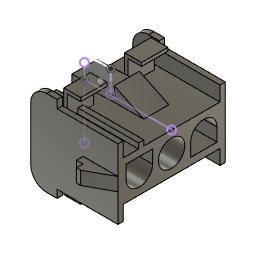
MLX_MF3_Connector_Mount (Autodesk Fusion 360 archive; units mm, degrees)
design "MLX Connector"
Autodesk Fusion 360 part; units mm, degrees
sketch "Sketch1" plane through (0, 0, 0) normal (1, 0, 0) x (0, 1, 0) in component "MLX Female Connector"
  line L0 (-10.15, 3.8) -> (-9.15, 3.8) construction
  line L1 (-9.15, -3.8) -> (-10.15, -3.8) construction
  line L2 (-10.15, -3.8) -> (-10.15, 3.8)
  line L3 (-10.15, 3.8) -> (-10.15, 6.6)
  line L4 (-10.15, 6.6) -> (-9.15, 6.6)
  line L5 (-9.15, 6.6) -> (-9.15, 3.8)
  line L6 (-10.15, -3.8) -> (-10.15, -6.6)
  line L7 (-10.15, -6.6) -> (-9.15, -6.6)
  line L8 (-9.15, -6.6) -> (-9.15, -3.8)
  line L9 (0, 3.8) -> (0, -3.8) construction
  line L10 (0, -3.8) -> (-9.15, -3.8)
  line L11 (-6.25, 3.8) -> (-5.25, 3.8)
  arc A0 (0, 2.5) -> (0, -2.5) centre (0, 0) ccw
  arc A1 (-8.6, 0) -> (-3.6, 0) centre (-6.1, 0) ccw
  line L12 (-3.6, 0) -> (-3.6, 2.5)
  line L13 (-3.6, 2.5) -> (-8.6, 2.5)
  line L14 (-8.6, 2.5) -> (-8.6, 0)
  line L15 (-6.25, 3.8) -> (-6.25, 4.8)
  line L16 (-6.25, 4.8) -> (-5.25, 4.8)
  line L17 (-5.25, 4.8) -> (-5.25, 3.8)
  line L18 (-5.25, 3.8) -> (0, 3.8)
  line L19 (-9.15, 3.8) -> (-6.25, 3.8)
  line L20 (5.25, 3.8) -> (0, 3.8)
  line L21 (6.25, 3.8) -> (5.25, 3.8)
  line L22 (0, -3.8) -> (9.15, -3.8)
  line L23 (9.15, -6.6) -> (9.15, -3.8)
  line L24 (10.15, -6.6) -> (9.15, -6.6)
  line L25 (10.15, -3.8) -> (10.15, -6.6)
  line L26 (10.15, -3.8) -> (10.15, 3.8)
  line L27 (10.15, 6.6) -> (9.15, 6.6)
  line L28 (9.15, 6.6) -> (9.15, 3.8)
  line L29 (10.15, 3.8) -> (10.15, 6.6)
  line L30 (9.15, 3.8) -> (6.25, 3.8)
  arc A2 (0, -2.5) -> (0, 2.5) centre (0, 0) ccw
  arc A3 (8.6, 0) -> (3.6, 0) centre (6.1, 0) ccw
  line L31 (3.6, 0) -> (3.6, -2.5)
  line L32 (3.6, -2.5) -> (8.6, -2.5)
  line L33 (8.6, -2.5) -> (8.6, 0)
  point P0 (10.15, 0)
  dimension "d4" = 7.6
  dimension "d5" = 1
  dimension "d6" = 2.8
  dimension "d7" = 10.15
  dimension "d8" = 2.5
  dimension "d9" = 2.5
  dimension "d10" = 6.1
  dimension "d11" = 1
  dimension "d12" = 1
  dimension "d13" = 4.9
  dimension "d15" = 6.1
  constraint horizontal L0
  constraint horizontal L1
  constraint vertical L2
  constraint vertical A0.centre L9.start
  constraint horizontal A0.centre P0
  constraint perpendicular L0 L3
  constraint perpendicular L3 L4
  constraint perpendicular L4 L5
  constraint perpendicular L1 L6
  constraint perpendicular L6 L7
  constraint perpendicular L1 L8
  constraint vertical L0.end L1.start
  constraint equal L3 L6
  constraint coincident L9.start L18.end
  constraint vertical L9
  constraint midpoint A0.centre L9
  constraint horizontal L10
  constraint horizontal L11
  constraint coincident L9 A0.end
  constraint coincident L9 A0.start
  constraint coincident A0.centre A2.centre
  constraint horizontal A1.start A1.end
  constraint horizontal A1.end A1.centre
  constraint horizontal A0.centre A1.centre
  constraint tangent A1 L12
  constraint perpendicular L12 L13
  constraint tangent A1 L14
  constraint tangent A0 L13
  constraint perpendicular L11 L15
  constraint perpendicular L15 L16
  constraint perpendicular L11 L17
  constraint horizontal L18
  constraint horizontal L19
  constraint symmetric L0.start L9 L26.end
  constraint symmetric L1.end L9 L25.start
  constraint symmetric L18.end L9 L20.end
  constraint symmetric L3.end L9 L27.start
  constraint symmetric L4.end L9 L27.end
  constraint symmetric L0.end L9 L28.end
  constraint symmetric L6.end L9 L24.start
  constraint symmetric L7.end L9 L23.start
  constraint symmetric L1.start L9 L22.end
  constraint symmetric L10.start L9 L22.start
  constraint symmetric L9 A0.start A2.end
  constraint symmetric L9 A0.end A2.start
  constraint symmetric L9 A0 A2
  constraint symmetric L9 L11.start L21.start
  constraint symmetric L9 L11.end L20.start
  constraint vertical L31
  constraint perpendicular L31 L32
  constraint perpendicular L32 L33
  constraint equal A1 A3
  constraint equal L12 L31
  constraint equal L31 L33
  constraint equal L13 L32
  constraint horizontal A1.centre A3.centre
  measures "d4" distance of L0.start L1.end
  measures "d5" distance of L3.end L4.end
  measures "d6" distance of L0.start L3.end
  measures "d7" distance of L2 L9
  measures "d8" radius of A0
  measures "d9" radius of A1
  measures "d10" horizontal distance of A0.centre A1.centre
  measures "d11" distance of L15.end L16.end
  measures "d12" distance of L11.start L15.end
  measures "d13" distance of L3 L17
  measures "d15" distance of A0.centre A3.centre
extrude "Extrude1" add sketch "Sketch1" along normal mid plane 16.5 in component "MLX Female Connector"
sketch "Sketch2" plane through (0, 0, 0) normal (0, 1, 0) x (1, 0, 0) in component "MLX Female Connector"
  line L0 (-8.25, -3.8) -> (8.25, -3.8)
  line L1 (8.25, -3.8) -> (-8.25, -3.8)
  line L2 (-8.25, -3.8) -> (-8.25, -5.9)
  line L3 (-8.25, -5.9) -> (0.001, -6.3012)
  line L4 (0.001, -6.3012) -> (-0.2312, -8)
  line L5 (-0.2312, -8) -> (5.35, -5.3)
  line L6 (5.35, -5.3) -> (0.001, -5.3)
  line L7 (0.001, -5.3) -> (-7.25, -4.9474)
  line L8 (-7.25, -4.9474) -> (-7.25, -3.8)
  line L9 (-8.25, 0) -> (8.25, 0) construction
  line L10 (-8.25, 3.8) -> (-8.25, 5.9)
  line L11 (-8.25, 5.9) -> (0.001, 6.3012)
  line L12 (0.001, 6.3012) -> (-0.2312, 8)
  line L13 (-0.2312, 8) -> (5.35, 5.3)
  line L14 (5.35, 5.3) -> (0.001, 5.3)
  line L15 (0.001, 5.3) -> (-7.25, 4.9474)
  line L16 (-7.25, 4.9474) -> (-7.25, 3.8)
  line L17 (8.25, 3.8) -> (-8.25, 3.8)
  dimension "d19" = 13.6
  dimension "d20" = 2.1
  dimension "d21" = 1
  dimension "d22" = 1
  dimension "d25" = 85
  dimension "d26" = 6.2
  dimension "d29" = 1.5
  dimension "d30" = 4.2
  constraint coincident L0.start L1.end
  constraint perpendicular L0 L2
  constraint parallel L3 L7
  constraint coincident L1 L8.end
  constraint perpendicular L1 L8
  constraint horizontal L6
  constraint vertical L3.end L6.end
  constraint parallel L0 L9
  constraint vertical L0.end L9.end
  constraint vertical L0.start L9.start
  constraint coincident origin L9
  constraint symmetric L0.start L9 L10.start
  constraint symmetric L0.end L9 L17.start
  constraint symmetric L2.end L9 L10.end
  constraint symmetric L3.end L9 L11.end
  constraint symmetric L4.end L9 L12.end
  constraint symmetric L5.end L9 L13.end
  constraint symmetric L6.end L9 L14.end
  constraint symmetric L7.end L9 L15.end
  constraint symmetric L8.end L9 L16.end
  measures "d19" distance of L2 L5.end
  measures "d20" distance of L0.start L2.end
  measures "d21" distance of L2 L8
  measures "d22" distance of L3 L7
  measures "d25" angle of L3 L4
  measures "d26" distance of L4.end L5.end
  measures "d29" distance of L0 L5.end
  measures "d30" distance of L1 L4.end
extrude "Extrude2" add sketch "Sketch2" along normal mid plane 4.75 in component "MLX Female Connector"
sketch "Sketch3" plane through (0, 0, 0) normal (0, 1, 0) x (1, 0, 0) in component "MLX Female Connector"
  line L0 (-8.25, -3.8) -> (-7.25, -3.8)
  line L1 (-7.25, -3.8) -> (-8.25, -3.8)
  line L2 (-8.25, -3.8) -> (8.25, -3.8)
  line L3 (8.25, -3.8) -> (-8.25, -3.8)
  line L4 (-3.9, -3.8) -> (-3.9, -8.75)
  line L5 (-3.9, -8.75) -> (-0.7, -8.75)
  line L6 (-0.7, -8.75) -> (-0.7, -8.1)
  line L7 (-0.7, -8.1) -> (-3.25, -8.1)
  line L8 (-3.25, -8.1) -> (-3.25, -3.8)
  line L9 (-3.9, -3.8) -> (-3.9, 0) construction
  line L10 (-3.9, 0) -> (8.25, 0) construction
  line L11 (8.25, 0) -> (8.25, -3.8) construction
  line L12 (-3.9, 3.8) -> (-3.9, 8.75)
  line L13 (-3.9, 8.75) -> (-0.7, 8.75)
  line L14 (-0.7, 8.75) -> (-0.7, 8.1)
  line L15 (-0.7, 8.1) -> (-3.25, 8.1)
  line L16 (-3.25, 8.1) -> (-3.25, 3.8)
  line L17 (-8.25, 3.8) -> (-7.25, 3.8)
  dimension "d33" = 0.65
  dimension "d34" = 0.65
  dimension "d35" = 3.2
  dimension "d36" = 4.95
  dimension "d42" = 12.15
  constraint perpendicular L0 L4
  constraint perpendicular L4 L5
  constraint perpendicular L5 L6
  constraint perpendicular L6 L7
  constraint coincident L1 L8.end
  constraint perpendicular L0 L8
  constraint perpendicular L0 L9
  constraint perpendicular L9 L10
  constraint coincident L2.end L3.start
  constraint perpendicular L3 L11
  constraint coincident origin L10
  constraint symmetric L0.start L10 L17.start
  constraint symmetric L0.end L10 L17.end
  constraint symmetric L4.start L10 L12.start
  constraint symmetric L4.end L10 L12.end
  constraint symmetric L5.end L10 L13.end
  constraint symmetric L6.end L10 L14.end
  constraint symmetric L7.end L10 L15.end
  constraint symmetric L8.end L10 L16.end
  constraint coincident L3 L4.start
  measures "d33" distance of L4 L8
  measures "d34" distance of L5 L7
  measures "d35" distance of L4.end L5.end
  measures "d36" distance of L4.start L4.end
  measures "d42" distance of L4 L2.end
extrude "Extrude3" add sketch "Sketch3" along normal blind 5 from surface at 3.25 in component "MLX Female Connector"
sketch "Sketch5" plane through (0, 0, 0) normal (0, 1, 0) x (1, 0, 0) in component "MLX Female Connector"
  line L0 (-3.25, -8.1) -> (-3.25, -3.8)
  line L1 (-8.25, 6.6) -> (-8.25, -6.6) construction
  line L2 (-8.25, -3.8) -> (8.25, -3.8)
  line L3 (-8.25, -3.8) -> (-8.25, -5.1)
  line L4 (-3.25, -8.1) -> (-5.25, -8.1)
  arc A0 (-8.25, -5.1) -> (-5.25, -8.1) centre (-5.25, -5.1) ccw
  line L5 (-8.25, -5.1) -> (-8.25, -8.1)
  line L6 (-8.25, -8.1) -> (-5.25, -8.1)
  dimension "d54" = 2
  constraint coincident L2.start L3.start
  constraint coincident L1 L3.end
  constraint perpendicular L2 L3
  constraint coincident L0.start L4.start
  constraint perpendicular L0 L4
  constraint tangent L1 A0
  constraint tangent L4 A0
  constraint tangent A0 L5
  constraint tangent A0 L6
  measures "d54" distance of L0.start L4.end
extrude "Extrude5" add sketch "Sketch5" along normal up to surface (1 mm away) from surface at 9.15 contours L0 L2 L3 L4 A0 in component "MLX Female Connector"
extrude "Extrude6" cut sketch "Sketch5" along normal up to surface (1 mm away) from surface at 9.15 contours A0 L5 L6 in component "MLX Female Connector"
mirror "Mirror1" about plane through (0, 0, 0) normal (0, 1, 0) of "Extrude3", "Extrude5", "Extrude6" in component "MLX Female Connector"
mirror "Mirror2" about plane through (0, 0, 0) normal (0, 0, 1) of "Extrude3", "Extrude5", "Extrude6", "Mirror1" in component "MLX Female Connector"
sketch "Sketch4" plane through (0, 0, 0) normal (0, 0, 1) x (1, 0, 0) in component "MLX Female Connector"
  line L0 (-3.25, 10.15) -> (8.25, 10.15)
  line L1 (8.25, 10.15) -> (3.6904, 12.65)
  line L2 (2.8904, 11.4) -> (1.65, 11.4)
  line L3 (1.65, 11.4) -> (1.65, 10.15)
  line L4 (3.6904, 12.65) -> (2.8904, 12.65)
  line L5 (2.8904, 12.65) -> (2.8904, 11.4)
  line L6 (-3.25, 10.15) -> (-3.25, 0) construction
  line L7 (-3.25, 0) -> (8.25, 0) construction
  line L8 (8.25, 0) -> (8.25, 10.15) construction
  line L9 (8.25, -10.15) -> (3.6904, -12.65)
  line L10 (3.6904, -12.65) -> (2.8904, -12.65)
  line L11 (2.8904, -12.65) -> (2.8904, -11.4)
  line L12 (2.8904, -11.4) -> (1.65, -11.4)
  line L13 (1.65, -11.4) -> (1.65, -10.15)
  line L14 (-3.25, -10.15) -> (8.25, -10.15)
  dimension "d45" = 2.5
  dimension "d46" = 1.25
  dimension "d47" = 6.6
  dimension "d48" = 5.2
  dimension "d49" = 0.8
  constraint coincident L0.end L1.start
  constraint coincident L0 L3.end
  constraint perpendicular L0 L3
  constraint horizontal L4
  constraint vertical L5
  constraint horizontal L2
  constraint coincident L0.start L6.start
  constraint perpendicular L0 L6
  constraint perpendicular L6 L7
  constraint perpendicular L0 L8
  constraint coincident origin L7
  constraint symmetric L0.start L7 L14.start
  constraint symmetric L0.end L7 L9.start
  constraint symmetric L1.end L7 L9.end
  constraint symmetric L2.start L7 L11.end
  constraint symmetric L2.end L7 L12.end
  constraint symmetric L3.end L7 L13.end
  constraint symmetric L4.end L7 L10.end
  measures "d45" vertical distance of L0.end L1.end
  measures "d46" distance of L0.end L2
  measures "d47" distance of L0.end L3
  measures "d48" distance of L0.end L1.end
  measures "d49" distance of L1.end L4.end
extrude "Extrude4" add sketch "Sketch4" along normal mid plane 2.5 in component "MLX Female Connector"
component "MLX Connector" placed x (1, 0, 0) y (0, 1, 0) z (0, 0, 1) at (0, 0, 0)
component "MLX Female Connector" placed x (1, 0, 0) y (0, 1, 0) z (0, 0, 1) at (0, 0, 0) in component "MLX Connector"
equation "molex_body_width = 20.3 mm"
equation "molex_body_height = 7.6 mm"
equation "d4 = molex_body_height"
equation "d6 = ( 13.2 mm - molex_body_height ) / 2"
equation "d7 = molex_body_width / 2"
equation "d8 = ( 5 / 2 ) * 1 mm"
equation "d9 = ( 5 / 2 ) * 1 mm"
equation "d10 = 1.1 mm + 5 mm"
equation "d12 = 8.6 mm - molex_body_height"
equation "d15 = 1.1 mm + 5 mm"
equation "molex_body_depth = 16.5 mm"
equation "d17 = molex_body_depth"
equation "d20 = ( 11.8 mm - molex_body_height ) / 2"
equation "d30 = ( 16 mm - molex_body_height ) / 2"
equation "d36 = ( 17.5 mm - molex_body_height ) / 2"
equation "d37 = ( 6.5 / 2 ) * 1 mm"
equation "d45 = ( 25.3 mm - molex_body_width ) / 2"
equation "d46 = ( 22.8 mm - molex_body_width ) / 2"
